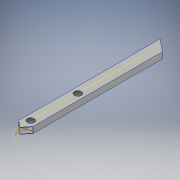
# Autodesk Inventor part: SUP_010_4BarBar
Saved by Autodesk Inventor 2018 (Build 220112000, 112)
## iProperties
Created: 2020-02-08
Part Number: SUP_010_4BarBar
Material: Aluminum 6061
Document SubType Name: Modeling
Designer: user
Mass: 267.937 g
Surface Area: 1262.16 cm^2
Volume: 99.236 cm^3
Density: 2.7 g/cm^3
Appearance: Aluminum - Flat
Author: user
Autodesk Inventor part; units mm, degrees
ref_plane "YZ Plane" through (0, 0, 0) normal (1, 0, 0) x (0, 1, 0)
ref_plane "XZ Plane" through (0, 0, 0) normal (0, 1, 0) x (-1, 0, 0)
ref_plane "XY Plane" through (0, 0, 0) normal (0, 0, 1) x (1, 0, 0)
sketch "Sketch1" plane through (0, 0, 0) normal (0, 0, 1) x (1, 0, 0)
  line L0 (0, 0) -> (50.8, 0)
  line L1 (50.8, 0) -> (50.8, 25.4)
  line L2 (50.8, 25.4) -> (0, 25.4)
  line L3 (0, 25.4) -> (0, 0)
  line L4 (1.5875, 1.5875) -> (49.2125, 1.5875)
  line L5 (49.2125, 1.5875) -> (49.2125, 23.8125)
  line L6 (49.2125, 23.8125) -> (1.5875, 23.8125)
  line L7 (1.5875, 23.8125) -> (1.5875, 1.5875)
  dimension "d0" = 50.8
  dimension "d1" = 25.4
  dimension "d2" = 1.5875
  constraints: 16 end point, 4 parallel, 2 perpendicular, 1 horizontal, 3 other
  measures "d0" distance of L2.end L1.end
  measures "d1" distance of L1.end L0.end
  measures "d2" distance between parallel lines of L3 L7
extrude "Extrusion1" add sketch "Sketch1" along normal blind 601.9292
sketch "Sketch2" plane through (0, 25.4, 0) normal (0, 1, 0) x (1, 0, 0)
  line L0 (125.8687, -681.3224) -> (26.7439, -601.9292)
  line L1 (26.7439, -601.9292) -> (85.6181, -528.4229)
  line L2 (85.6181, -528.4229) -> (184.7429, -607.8161)
  line L3 (184.7429, -607.8161) -> (125.8687, -681.3224)
  line L4 (-52.6493, -701.054) -> (26.7439, -601.9292)
  line L5 (26.7439, -601.9292) -> (-41.6165, -547.1765)
  line L6 (-41.6165, -547.1765) -> (-121.0097, -646.3013)
  line L7 (-121.0097, -646.3013) -> (-52.6493, -701.054)
  line L8 (50.8, 0) -> (0, 0) projected
  line L9 (0, 0) -> (0, -601.9292) projected
  line L10 (50.8, -601.9292) -> (0, -601.9292) projected
  line L11 (50.8, 0) -> (50.8, -601.9292) projected
  line L12 (0, 0) -> (0, -601.9292) projected
  point P0 (50.8, -571.8944)
  point P1 (0, -580.5089)
  dimension "d6" = 127
  dimension "d7" = 127
  dimension "d9" = 38.481
  dimension "d16" = 34.2646
  constraints: 16 end point, 5 parallel, 5 point on line, 2 perpendicular
  measures "d6" distance of L4.start L0.end
  measures "d7" distance of L1.end L2.end
  measures "d9" distance of point (50.8, -571.894) L0.end
  measures "d16" distance from line of L4 point (0, -580.509)
extrude "Extrusion2" cut sketch "Sketch2" against normal blind 25.4 contours L0 L10 L11 L1 L2 L3 | L10 L9 L5 | L1 L11 L10 | L4 L7 L6 L5 L9 L10
sketch "Sketch3" plane through (0, 25.4, 0) normal (0, 1, 0) x (1, 0, 0)
  line L0 (0, 0) -> (59.8042, 74.6674)
  line L1 (59.8042, 74.6674) -> (161.4042, -6.7083)
  line L2 (161.4042, -6.7083) -> (101.6, -81.3757)
  line L3 (101.6, -81.3757) -> (0, 0)
  line L4 (50.8, 0) -> (0, 0) projected
  line L5 (50.8, 0) -> (50.8, -571.8944) projected
  line L6 (0, -580.5089) -> (26.7439, -601.9292) projected
  point P0 (50.8, -40.6878)
  constraints: 8 end point, 3 parallel, 1 midpoint, 1 perpendicular, 1 point on line
extrude "Extrusion3" cut sketch "Sketch3" against normal blind 25.4 contours L4 L5 L3
sketch "Sketch4" plane through (0, 25.4, 580.5089) normal (0, 1, 0) x (1, 0, 0)
  line L0 (-37.1172, 580.5089) -> (145.2482, 580.5089) construction
  line L1 (0, 580.5089) -> (0, 0) construction
  point P0 (25.4, 217.3651)
  point P1 (25.4, 24.1981)
  point P2 (26.7439, -21.4203)
  dimension "d17" = 25.4
  dimension "d20" = 25.4
  dimension "d28" = 238.7854
  dimension "d29" = 45.6184
  constraints: 2 end point, 1 horizontal, 1 point on line
  measures "d17" distance from line of L1 point (25.4, 217.365)
  measures "d20" distance from line of L1 point (25.4, 24.198)
  measures "d28" vertical distance of point (25.4, 217.365) point (26.744, -21.42)
  measures "d29" vertical distance of point (26.744, -21.42) point (25.4, 24.198)
hole "Hole1" at (25.4, 25.4, 363.1438) at (25.4, 25.4, 556.3108) direction (0, -1, 0) diameter 28.575 depth 25.4 tip angle 118
ref_plane "Work Plane1" through (25.4, 0, 571.8944) normal (1, 0, 0) x (0, 0, -1)
body "Solid1"
